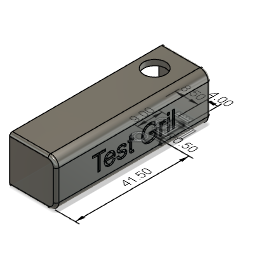
PacifierVape (Autodesk Fusion 360 design; units mm, degrees)
Autodesk Fusion 360 part; units mm, degrees
sketch "Sketch1" plane through (0, 0, 0) normal (0, 0, 1) x (1, 0, 0)
  line L0 (0, 0) -> (14, 0)
  line L1 (17, 3) -> (17, 14)
  line L2 (14, 17) -> (0, 17)
  line L3 (0, 17) -> (0, 0)
  arc A0 (17, 14) -> (14, 17) centre (14, 14) ccw
  arc A1 (14, 0) -> (17, 3) centre (14, 3) ccw
  line L4 (0, 0) -> (17, 0)
  line L5 (17, 0) -> (17, 17)
  line L6 (17, 17) -> (0, 17)
  line L7 (0, 17) -> (0, 0)
  point P0 (17, 0)
  point P1 (17, 17)
  dimension "d1" = 17
  dimension "d2" = 17
  dimension "d5" = 3
  constraint horizontal L0
  constraint vertical L1
  constraint horizontal L2
  constraint vertical L3
  constraint coincident L0.start L3.end
  constraint coincident P1 L1
  constraint coincident P1 L2
  constraint tangent L1 A0
  constraint tangent L2 A0
  constraint coincident P0 L0
  constraint coincident P0 L1
  constraint tangent L0 A1
  constraint tangent L1 A1
  constraint equal A0 A1
  constraint horizontal L4
  constraint vertical L5
  constraint horizontal L6
  constraint vertical L7
  constraint coincident P1 L5.end
  measures "d1" distance of L1 L3
  measures "d2" distance of P0 P1
  measures "d5" radius of A1
extrude "Extrude1" add sketch "Sketch1" along normal blind 56.5 contours L0 L1 L2 L3 A0 A1 L4 L5 L6 L7
sketch "Button" plane through (0, 17, 0) normal (0, 1, 0) x (-1, 0, 0)
  line L0 (-14, 0) -> (0, 0)
  line L1 (0, 0) -> (0, 56.5)
  line L2 (0, 56.5) -> (-14, 56.5)
  line L3 (-14, 56.5) -> (-14, 0)
  circle A0 centre (-6, 9.5) radius 4
  dimension "d8" = 8
  dimension "d9" = 6
  dimension "d10" = 47
  measures "d8" diameter of A0
  measures "d9" distance of L1 A0.centre
  measures "d10" distance of L2 A0.centre
shell "Shell1" thickness 2 removed faces 1 at (0, 11.3333, 18.8333)
extrude "Extrude2" cut sketch "Button" against normal blind 3 contours A0
fillet "Fillet1" radius 1 10 edges at (7, 0, 0) (16.1213, 0.8787, 0) (17, 8.5, 0) (16.1213, 16.1213, 0) (7, 17, 0) (7, 0, 56.5) (16.1213, 0.8787, 56.5) (17, 8.5, 56.5) (16.1213, 16.1213, 56.5) (7, 17, 56.5)
sketch "Text" plane through (17, 0, 0) normal (1, 0, 0) x (0, 0, -1)
  line L0 (-55.5, 14) -> (-55.5, 3)
  line L1 (-55.5, 3) -> (-1, 3)
  line L2 (-1, 3) -> (-1, 14)
  line L3 (-1, 14) -> (-55.5, 14)
  line L4 (-55.5, 3) -> (-1, 3) construction
  line L5 (-1, 3) -> (-1, 14) construction
  line L6 (-1, 14) -> (-55.5, 14) construction
  line L7 (-55.5, 14) -> (-55.5, 3) construction
  dimension "d16" = 6
  text T0 "Test Gril" font "Arial" height 6 align centre middle in box 54.5 x 11 at (-55.5, 3) x (1, 0) y (0, 1) spacing 1 kerned
  constraint coincident L2.end
  constraint coincident L0.end
extrude "Extrude3" cut sketch "Text" against normal blind 0.5 text T0
sketch "Sketch4" plane through (0, 0, 0) normal (0, -1, 0) x (1, 0, 0)
  line L0 (14, 55.5) -> (0, 55.5)
  line L1 (0, 55.5) -> (0, 1)
  line L2 (0, 1) -> (14, 1)
  line L3 (14, 1) -> (14, 55.5)
  line L4 (8.5, 5) -> (12, 5)
  line L5 (12.5, 5.5) -> (12.5, 13.5)
  line L6 (12, 14) -> (8.5, 14)
  line L7 (8.5, 14) -> (8.5, 5)
  arc A0 (12.5, 13.5) -> (12, 14) centre (12, 13.5) ccw
  arc A1 (12, 5) -> (12.5, 5.5) centre (12, 5.5) ccw
  dimension "d20" = 9
  dimension "d21" = 8.5
  dimension "d24" = 0.5
  dimension "d26" = 41.5
  dimension "d27" = 4
  constraint horizontal L4
  constraint vertical L5
  constraint horizontal L6
  constraint vertical L7
  constraint tangent L5 A0
  constraint tangent L6 A0
  constraint tangent L4 A1
  constraint tangent L5 A1
  constraint equal A0 A1
  measures "d20" distance of L4.start L6.end
  measures "d21" distance of L1 L7
  measures "d24" radius of A0
  measures "d26" distance of L0 L6
  measures "d27" distance of L5 L7
extrude "Extrude4" [rolled back] along distance -3 taper angle 0
